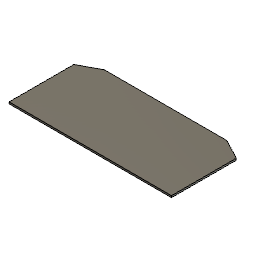
lid (Autodesk Fusion 360 design; units mm, degrees)
Autodesk Fusion 360 part; units mm, degrees
sketch "Sketch1" plane through (0, 0, 0) normal (0, 1, 0) x (1, 0, 0)
  line L0 (0, -265) -> (570, -265)
  line L1 (0, -37.5) -> (70, 0)
  line L2 (570, -37.5) -> (500, 0)
  line L3 (0, -37.5) -> (0, -265)
  line L4 (70, 0) -> (500, 0)
  line L5 (570, -37.5) -> (570, -265)
  dimension "d2" = 265
  dimension "d6" = 37.5
  constraint perpendicular L0 L3
  constraint perpendicular L3 L4
  constraint perpendicular L4 L5
  measures "d2" distance of origin L0.start
  measures "d6" distance of origin L1.start
extrude "Extrude1" add sketch "Sketch1" along normal blind 6.35
